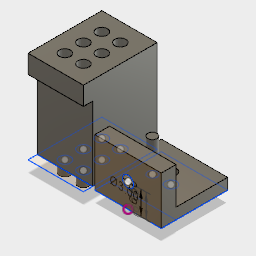
line follower v1 (Autodesk Fusion 360 design; units mm, degrees)
Autodesk Fusion 360 part; units mm, degrees
sketch "Sketch1" plane through (0, 0, 0) normal (0, 1, 0) x (1, 0, 0)
  line L0 (0.1507, -0.0574) -> (18.1507, -0.0574)
  line L1 (18.1507, -0.0574) -> (18.1507, -18.0574)
  line L2 (18.1507, -18.0574) -> (0.1507, -18.0574)
  line L3 (0.1507, -18.0574) -> (0.1507, -0.0574)
  circle A0 centre (9.1507, -6.4574) radius 1.5
  line L4 (0.1507, -18.0574) -> (18.1507, -18.0574)
  line L5 (18.1507, -18.0574) -> (18.1507, -14.0574)
  line L6 (18.1507, -14.0574) -> (0.1507, -14.0574)
  line L7 (0.1507, -14.0574) -> (0.1507, -18.0574)
  circle A1 centre (4.2507, -6.5574) radius 1.25
  dimension "d4" = 18
  dimension "d5" = 18
  dimension "d6" = 3
  dimension "d7" = 9
  dimension "d9" = 4
  dimension "d27" = 2.5
  dimension "d28" = 4.9
  dimension "d35" = 7.6
  dimension "d36" = 7.5
  measures "d4" distance of L1 L3
  measures "d5" distance of L0 L2
  measures "d6" diameter of A0
  measures "d7" distance of L3 A0.centre
  measures "d9" distance of L4 L6
  measures "d27" diameter of A1
  measures "d28" distance of A0.centre A1.centre
  measures "d35" distance of A0.centre L6
  measures "d36" distance of L6 A1.centre
extrude "Extrude1" add sketch "Sketch1" along normal blind 3 contours L0 L1 L3 L6 | A1 makes body 1
extrude "Extrude2" add sketch "Sketch1" along normal blind 13 contours L1 L2 L3 L4 L5 L6 L7 bodies 1
sketch "Sketch2" plane through (0, 0, 18.0574) normal (0, 0, 1) x (1, 0, 0)
  line L0 (0.1507, 0) -> (18.1507, 0)
  line L1 (18.1507, 0) -> (18.1507, 13)
  line L2 (18.1507, 13) -> (0.1507, 13)
  line L3 (0.1507, 13) -> (0.1507, 0)
  circle A0 centre (9.1507, 6.5) radius 1.5
  point P0 (9.1507, 0)
  dimension "d25" = 6.5
  dimension "d26" = 7
  dimension "d33" = 3
  measures "d25" distance of A0.centre P0
  measures "d33" diameter of A0
extrude "Extrude4" cut sketch "Sketch2" along normal mid plane 20 contours A0 bodies 1
extrude "Extrude6" add sketch "Sketch1" along normal blind 9 separate body contours A1 makes body 2
sketch "Sketch3" plane through (0, 0, 0) normal (0, 1, 0) x (1, 0, 0)
  line L0 (-16, 0) -> (-1, 0)
  line L1 (-1, 0) -> (-1, -20)
  line L2 (-1, -20) -> (-16, -20)
  line L3 (-16, -20) -> (-16, 0)
  circle A0 centre (-11, -5) radius 1.5
  circle A1 centre (-6, -5) radius 1.5
  circle A2 centre (-11, -10) radius 1.5
  circle A3 centre (-6, -10) radius 1.5
  circle A4 centre (-11, -15) radius 1.5
  circle A5 centre (-6, -15) radius 1.5
  line L4 (-16, -17.5) -> (-1, -17.5)
  line L5 (-1, -17.5) -> (-1, -20)
  line L6 (-1, -20) -> (-16, -20)
  line L7 (-16, -20) -> (-16, -17.5)
  dimension "d37" = 15
  dimension "d38" = 20
  dimension "d39" = 3
  dimension "d40" = 5
  dimension "d41" = 5
  dimension "d42" = 3
  dimension "d43" = 5
  dimension "d44" = 3
  dimension "d45" = 3
  dimension "d46" = 5
  dimension "d47" = 5
  dimension "d48" = 5
  dimension "d49" = 5
  dimension "d50" = 3
  dimension "d51" = 3
  dimension "d52" = 5
  dimension "d53" = 5
  dimension "d54" = 5
  dimension "d55" = 5
  dimension "d56" = 5
  dimension "d57" = 7.5
  measures "d37" distance of L0.start L0.end
  measures "d38" distance of L0 L2
  measures "d39" diameter of A0
  measures "d40" distance of L0 A0.centre
  measures "d41" distance of L3 A0.centre
  measures "d42" diameter of A1
  measures "d43" distance of A0.centre A1.centre
  measures "d44" diameter of A2
  measures "d45" diameter of A3
  measures "d46" distance of A2.centre A3.centre
  measures "d47" distance of A0.centre A2.centre
  measures "d48" distance of A1.centre A3.centre
  measures "d49" distance of L0 A1.centre
  measures "d50" diameter of A4
  measures "d51" diameter of A5
  measures "d52" distance of A2.centre A4.centre
  measures "d53" distance of A3.centre A5.centre
  measures "d54" distance of A4.centre A5.centre
  measures "d55" distance of L3 A4.centre
  measures "d56" distance of L3 A2.centre
  measures "d57" distance of A3.centre L4
extrude "Extrude7" add sketch "Sketch3" along normal blind 25 separate body contours L0 L1 L3 L4 makes body 3
extrude "Extrude8" add sketch "Sketch3" along normal blind 5 from surface at 20 contours L1 L2 L3 L4 L5 L6 L7 bodies 3
extrude "Extrude9" add sketch "Sketch3" against normal blind 3 separate body contours A0 | A1 | A4 | A5 makes body 4 at (-4.5019, -2, 5.0748) makes body 5 at (-4.5019, -2, 15.0748) makes body 6 at (-9.5019, -2, 5.0748) makes body 7 at (-9.5019, -2, 15.0748)
copy_body "CutPasteBodies1" bodies 3 4 5 6 7 removing the originals makes body 8 makes body 9 makes body 10 makes body 11 makes body 12 in component "Component"
component "Component" placed x (1, 0, 0) y (0, 1, 0) z (0, 0, 1) at (0, 0, 0)
